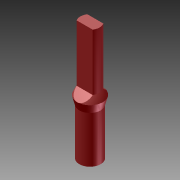
# Autodesk Inventor part: tl5CC-17.5mmtoggle
Saved by Autodesk Inventor 2011 SP1 (Build 150282100, 282)
## iProperties
Created: 2013-12-24
Part Number: tl5CC-17.5mmtoggle
Catalog Web Link: www.cadenas.de
Description: TL Series - Fully Illuminated Toggles - 17.5 mm toggle-
Vendor: NKKSWITCHES
Document SubType Name: Modeling
Designer: PARTuser1
Manufacturer: NKKSWITCHES
Density: 1 g/cm^3
Category: PARTsolutions
Company: NKKSWITCHES
Title: tl5CC-17.5mmtoggle
Author: Cadenas PARTsolutions
PSOL_IDENT_0: {$CADENAS_DATA\23d-libs\nkkswitches\toggle\tl\parts\tl_toggle_17.prj},231 {VTYP=3D},{NB=tl5CC-17.5mm
PSOL_IDENT_1: toggle},{LINA=tl5CC-17.5mmtoggle},{NN=TL Series - Fully Illuminated Toggles - 17.5 mm toggle},{DATE=
PSOL_IDENT_2: 08.04.2009 12:11:38},{GEOMDATE=26.03.2009 00:00:00},{VERSION=},{LINEID=10},{LINESUBID=-1},{WBVAR=TC,
PSOL_IDENT_3: LC}  {NB=tl5CC-17.5mmtoggle},{LINA=tl5CC-17.5mmtoggle},{KT=DUMMY},{SRS=TL},{PN=tl5CC-17.5mmtoggle},{
PSOL_IDENT_4: TC=C},{COLOR=RED},{COLORALG=1.00,0.00,0.00,0.00},{LC=5C},{LCALG= '5C', 'Red' }
CNS_NN: TL Series - Fully Illuminated Toggles - 17.5 mm toggle
CNS_NB: tl5CC-17.5mmtoggle
CNS_NBSYN: $PN.
CNS_LINA: tl5CC-17.5mmtoggle
CNS_SRS: TL
CNS_PN: tl5CC-17.5mmtoggle
CNS_TC: Red
CNS_COLOR: RED
CNS_COLORALG: 1.00,0.00,0.00,0.00
CNS_LC: Red
CNS_LCALG: '5C', 'Red'
SUPPLIER: NKKSWITCHES
ARTICLENO: tl5CC-17.5mmtoggle
BOMINFO: tl5CC-17.5mmtoggle
CREATOR: CADENAS GmbH
Autodesk Inventor part; units mm, degrees
sketch "Sketch_1" plane through (0, 0, 0) normal (0, 0, 1) x (1, 0, 0)
  line L0 (0, 17.5006) -> (0, -10.0076)
  line L1 (0, -10.0076) -> (-2.4892, -10.0076)
  line L2 (-2.4892, -10.0076) -> (-2.4892, 0.8636)
  line L3 (-2.4892, 0.8636) -> (-2.9972, 2.7813)
  arc A0 (-2.2479, 4.3053) -> (-2.9972, 2.7813) centre (6.4631, -0.9238) ccw
  line L4 (-2.2479, 4.3053) -> (-2.2479, 17.5006)
  line L5 (-2.2479, 17.5006) -> (0, 17.5006)
  line L6 (0, 17.5006) -> (0, -10.0076)
  constraints: 14 end point, 2 point on circle, 1 centre point
revolve "Revolution1" add sketch "Sketch_1" angle 360 about axis through (0, 17.5006, 0) along (0, 1, 0)
sketch "Sketch_2" plane through (0, 0, 0) normal (1, 0, 0) x (0, 1, 0)
  line L0 (18.7706, 4.0132) -> (0.9906, 4.0132)
  line L1 (0.9906, 4.0132) -> (0.9906, 2.9972)
  line L2 (0.9906, 2.9972) -> (2.7686, 2.9972)
  line L3 (2.7686, 2.9972) -> (4.2926, 1.2446)
  line L4 (4.2926, 1.2446) -> (18.0086, 1.2446)
  line L5 (18.0086, 1.2446) -> (18.0086, -1.2446)
  line L6 (18.0086, -1.2446) -> (4.2926, -1.2446)
  line L7 (4.2926, -1.2446) -> (2.7686, -2.9972)
  line L8 (2.7686, -2.9972) -> (0.9906, -2.9972)
  line L9 (0.9906, -2.9972) -> (0.9906, -4.0132)
  line L10 (0.9906, -4.0132) -> (18.7706, -4.0132)
  line L11 (18.7706, -4.0132) -> (18.7706, 4.0132)
  constraints: 24 end point
extrude "Extrusion1" cut sketch "Sketch_2" along normal mid plane 5.08
ref_plane "toggle17_5_to_body_XY" through (0, 0, 0.254) normal (0, 1, 0) x (1, 0, 0)
ref_plane "toggle17_5_to_body_YZ" through (0, 0, 0.254) normal (1, 0, 0) x (0, 0, -1)
ref_plane "toggle17_5_to_body_ZX" through (0, 0, 0.254) normal (0, 0, -1) x (0, 1, 0)
body "Solid1"
